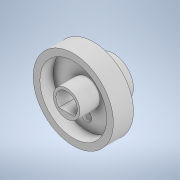
# Autodesk Inventor part: spoolEPN
Saved by Autodesk Inventor 2021 (Build 250183000, 183)
## iProperties
Created: 2021-07-20
Part Number: spoolEPN
Material: Generic
Document SubType Name: Modeling
Designer: ztjona!
Density: 1 g/cm^3
Appearance: Default
Author: ztjona!
Autodesk Inventor part; units mm, degrees
ref_plane "YZ Plane" through (0, 0, 0) normal (1, 0, 0) x (0, 1, 0)
ref_plane "XZ Plane" through (0, 0, 0) normal (0, 1, 0) x (-1, 0, 0)
ref_plane "XY Plane" through (0, 0, 0) normal (0, 0, 1) x (1, 0, 0)
sketch "Sketch1" plane through (0, 0, 0) normal (0, 0, 1) x (1, 0, 0)
  arc A0 (0.8307, -1) -> (-0.8307, -1) centre (0, 0) ccw projected
  line L0 (-0.8307, -1) -> (0.8307, -1) projected
  arc A1 (1.118, -1) -> (-1.118, -1) centre (0, 0) ccw projected
  line L1 (-1.118, -1) -> (-0.8307, -1) projected
  line L2 (0.8307, -1) -> (1.118, -1) projected
  line L3 (-0.8307, -1.1) -> (-1.1619, -1.1)
  arc A2 (1.1619, -1.1) -> (-1.1619, -1.1) centre (0, 0) ccw
  line L4 (1.1619, -1.1) -> (0.8307, -1.1)
  line L5 (-0.8307, -1.1) -> (0.8307, -1.1)
  circle A3 centre (0, 0) radius 2
  dimension "d0" = 0.1
  dimension "d1" = 4
  constraints: 6 end point, 2 centre point, 2 point on circle, 1 coincident, 1 horizontal, 2 other
  measures "d0" radial gap between concentric circles of A1 A2
  measures "d1" diameter of A3
extrude "Extrusion1" add sketch "Sketch1" against normal blind 2.5 contours A3
sketch "Sketch2" plane through (0, 0, -2.5) normal (0, 0, -1) x (-1, 0, 0)
  circle A0 centre (0, 0) radius 2 projected
  line L0 (1.1619, -1.1) -> (-1.1619, -1.1) projected
  arc A1 (1.1619, -1.1) -> (-1.1619, -1.1) centre (0, 0) ccw projected
  circle A2 centre (0, 0) radius 6
  dimension "d4" = 12
  constraints: 1 centre point, 1 coincident
  measures "d4" diameter of A2
extrude "Extrusion2" add sketch "Sketch2" along normal blind 1.5 contours A0 | A2
sketch "Sketch3" plane through (0, 0, -4) normal (0, 0, -1) x (-1, 0, 0)
  circle A0 centre (0, 0) radius 6 projected
  line L0 (1.1619, -1.1) -> (-1.1619, -1.1) projected
  arc A1 (1.1619, -1.1) -> (-1.1619, -1.1) centre (0, 0) ccw projected
  circle A2 centre (0, 0) radius 3
  dimension "d7" = 6
  constraints: 1 centre point, 1 coincident
  measures "d7" diameter of A2
extrude "Extrusion3" add sketch "Sketch3" along normal blind 3 contours A2
sketch "Sketch4" plane through (0, 0, -7) normal (0, 0, -1) x (-1, 0, 0)
  circle A0 centre (0, 0) radius 6
  circle A1 centre (0, 0) radius 3 projected
  circle A2 centre (0, 0) radius 6 projected
  circle A3 centre (0, 0) radius 3 projected
  line L0 (1.1619, -1.1) -> (-1.1619, -1.1) projected
  arc A4 (1.1619, -1.1) -> (-1.1619, -1.1) centre (0, 0) ccw projected
  constraints: 1 centre point, 1 coincident, 1 concentric
extrude "Extrusion4" add sketch "Sketch4" along normal blind 1.5 contours A0 | A1
sketch "Sketch5" plane through (0, 0, -2.5) normal (0, 0, 1) x (1, 0, 0)
  circle A0 centre (0, 0) radius 6 projected
  circle A1 centre (0, 0) radius 2 projected
  circle A2 centre (0, 0) radius 2 projected
  circle A3 centre (0, 0) radius 2 projected
  line L0 (1.1619, -1.1) -> (-1.1619, -1.1) projected
  arc A4 (1.1619, -1.1) -> (-1.1619, -1.1) centre (0, 0) ccw projected
  circle A5 centre (0, 0) radius 5
  dimension "d12" = 1
  constraints: 1 centre point, 1 coincident
  measures "d12" radial gap between concentric circles of A0 A5
extrude "Extrusion5" add sketch "Sketch5" along normal up to surface (2.5 mm away) contours A0
sketch "Sketch6" plane through (0, 0, -2.5) normal (0, 0, 1) x (1, 0, 0)
  circle A0 centre (0, 0) radius 2 projected
  line L0 (1.1619, -1.1) -> (-1.1619, -1.1) projected
  arc A1 (1.1619, -1.1) -> (-1.1619, -1.1) centre (0, 0) ccw projected
  circle A2 centre (0, 0) radius 5 projected
  circle A3 centre (0, 0) radius 2 projected
  circle A4 centre (0, 0) radius 5 projected
  circle A5 centre (0, 0) radius 6 projected
  circle A6 centre (0, 0) radius 3 projected
  circle A7 centre (0, -3.15) radius 0.75
  line L1 (-8.4, 0) -> (8.4, 0) projected
  line L2 (-0.5604, -2.4) -> (0.7136, -2.4) construction
  line L3 (-0.4416, -3) -> (0.9927, -3) construction
  line L4 (0, -8.4) -> (0, 8.4) projected
  point P0 (0, -3.9)
  dimension "d16" = 1.5
  dimension "d25" = 0.6
  constraints: 4 end point, 2 horizontal, 2 point on line, 1 tangent, 1 vertical alignment, 2 other
  measures "d25" distance between parallel lines of L2 L3
extrude "Extrusion6" cut sketch "Sketch6" against normal blind 1.8 contours L4 A6 A7 | A7 A6 L4 | A7 L4 A6 | A6 L4 A7
move faces "Move1" translate (0, 0, -1) faces at (5.5601, -0.8775, 0)
move faces "Move2" translate (0, 0, -0.5) faces at (3.9516, -0.3989, -2.5)
move faces "Move3" translate (0, 0, 1.5) faces at (-0.2411, -2.7188, -8.5)
body "Solid1"
